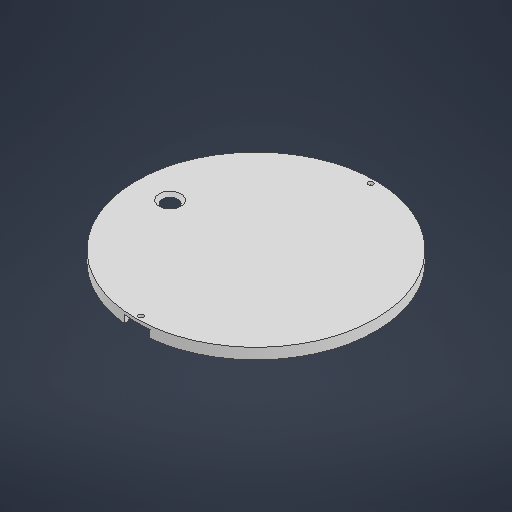
# Autodesk Inventor part: Vial Cover
Saved by Autodesk Inventor 2025.1 (Build 291241000, 241)
## iProperties
Created: 2025-02-24
Part Number: Vial Cover
Material: Generic
Document SubType Name: Modeling
Designer: jerem
Density: 1 g/cm^3
Appearance: Default
Author: jerem
## iProperties of the stored document Vial Cover_3DPrint.ipt
Created: 2025-02-24
Part Number: Vial Cover_3DPrint
Material: Generic
Document SubType Name: Modeling
Designer: jerem
Density: 1 g/cm^3
Appearance: Default
Author: jerem
Autodesk Inventor part; units mm, degrees
ref_plane "YZ Plane" through (0, 0, 0) normal (1, 0, 0) x (0, 1, 0)
ref_plane "XZ Plane" through (0, 0, 0) normal (0, 1, 0) x (-1, 0, 0)
ref_plane "XY Plane" through (0, 0, 0) normal (0, 0, 1) x (1, 0, 0)
sketch "Sketch1" plane through (0, 0, 0) normal (0, 1, 0) x (-1, 0, 0)
  circle A0 centre (0, 0) radius 70.5
  circle A1 centre (55, 0) radius 5
  line L0 (55, 0) -> (0, 0) construction
  line L1 (0, 0) -> (0, 70.5) construction
  circle A2 centre (0, 0) radius 76.5
  circle A3 centre (0, 73.5) radius 1.6
  line L2 (0, 73.5) -> (0, 70.5) construction
  line L3 (8.2, 76.0593) -> (8.2, 70.0215)
  line L4 (-8.2, 76.0593) -> (-8.2, 70.0215)
  line L5 (8.2, 70.0215) -> (-8.2, 70.0215) construction
  circle A4 centre (0, -73.5) radius 1.6
  line L6 (0, -73.5) -> (0, -70.5) construction
  line L7 (8.2, -76.0593) -> (8.2, -70.0215)
  line L8 (-8.2, -76.0593) -> (-8.2, -70.0215)
  line L9 (8.2, -70.0215) -> (-8.2, -70.0215) construction
  point P0 (-8.2, -70.0215)
  point P1 (-8.2, -76.0593)
  point P2 (8.2, -76.0593)
  point P3 (8.2, -70.0215)
  dimension "d0" = 141
  dimension "d1" = 10
  dimension "d2" = 55
  dimension "d8" = 6
  dimension "d9" = 3.2
  dimension "d10" = 3
  dimension "d11" = 16.4
  constraints: 20 end point, 6 symmetric about line, 5 centre point, 5 point on circle, 4 vertical, 2 coincident, 2 horizontal, 1 other
  measures "d0" diameter of A0
  measures "d1" diameter of A1
  measures "d2" distance of L0.start L0.end
  measures "d8" radial gap between concentric circles of A0 A2
  measures "d9" diameter of A3
  measures "d10" distance of L2.start L1.end
  measures "d11" distance of L3.end L4.end
extrude "Extrusion1" add sketch "Sketch1" along normal blind 2
chamfer "Chamfer1" distance 2 angle 45 1 edges at (-50, 2, 0)
extrude "Extrusion2" add sketch "Sketch1" against normal blind 5 contours A0 L3 A2 L7 | A0 L8 A2 L4
chamfer "Chamfer3" distance 4 distance2 5 1 edges at (-70.5, -5, 0) measured on face at (-71, -5, 0)
chamfer "Chamfer4" distance 4 distance2 5 1 edges at (70.5, -5, 0) measured on face at (71, -5, 0)
body "Solid1"
